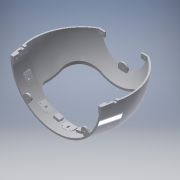
# Autodesk Inventor part: front
Saved by Autodesk Inventor 2017 (Build 210142000, 142)
## iProperties
Part Number: front
Material: Genérico
Document SubType Name: Modeling
Designer: Roberto
Density: 1 g/cm^3
Appearance: Valor por defecto
Author: Roberto
Autodesk Inventor part; units mm, degrees
ref_plane "XY Plane" through (0, 0, 0) normal (0, 0, 1) x (1, 0, 0)
sketch "Boceto1" plane through (0, 0, 0) normal (0, 0, 1) x (1, 0, 0)
  line L0 (-0.611288, 3.290752) -> (-0.374025, 3.347948)
  line L1 (0.276744, 0) -> (-0.374025, 3.347948)
  line L2 (-0.374025, 3.347945) -> (0.276744, 0)
  line L3 (-0.611288, 3.290752) -> (0, 0)
  line L4 (-0.611288, 3.290752) -> (0, 0)
  line L5 (0, 0) -> (0.3056, 0)
  line L6 (0.276744, 0) -> (0, 0)
  line L7 (0, 0) -> (0.3056, 0)
  line L8 (0, 0) -> (15, 0)
  arc A0 (3.961812, 11.346952) -> (-0.374025, 3.347948) centre (7.685812, 4.153752) ccw
  arc A1 (7.5, 12.385014) -> (3.894598, 11.311754) centre (8.396412, 2.781252) ccw
  line L9 (7.5, 12.627938) -> (7.5, 12.385014)
  arc A2 (7.5, 12.627938) -> (3.850449, 11.561628) centre (8.396412, 2.781252) ccw
  arc A3 (3.850449, 11.561628) -> (-0.611288, 3.290752) centre (7.685812, 4.153752) ccw
  line L10 (7.5, 0) -> (7.5, 18.610852)
  dimension "d0" = 15
  constraints: 22 end point, 11 point on circle, 4 centre point, 3 collinear, 3 horizontal, 2 coincident, 2 vertical, 1 midpoint
  measures "d0" distance of L5.start L8.end
revolve "Revolución1" add sketch "Boceto1" angle 180 about axis through (7.5, 12.627938, 0) along (0, -1, 0) contours A3 A2 L9 A1 A0 L0 | L0 L1 L5 L3
sketch "Boceto2" plane through (7.5, 0, 0) normal (0, -1, 0) x (1, 0, 0)
  circle A0 centre (-4.734, 4.734) radius 0.15
  circle A1 centre (4.734, 4.734) radius 0.15
  arc A2 (7.5, 0) -> (-7.5, 0) centre (0, 0) ccw
  arc A3 (-5.19458, 4.349466) -> (-4.349466, 5.19458) centre (-4.734, 4.734) ccw
  line L0 (-4.27342, 5.118534) -> (-4.763502, 5.608616)
  line L1 (-5.118534, 4.273421) -> (-5.611701, 4.766588)
  line L2 (0, 0) -> (0, 11.293859)
  circle A4 centre (4.734, 4.734) radius 0.15
  arc A5 (7.5, 0) -> (-7.5, 0) centre (0, 0) ccw
  arc A6 (4.349466, 5.19458) -> (5.19458, 4.349466) centre (4.734, 4.734) ccw
  line L3 (4.27342, 5.118534) -> (4.863883, 5.708997)
  line L4 (5.118534, 4.273421) -> (5.610829, 4.765715)
  line L5 (-4.663121, 5.508235) -> (-4.763502, 5.608616)
  line L6 (-5.514406, 4.669292) -> (-5.611701, 4.766588)
  line L7 (-5.611701, 4.766588) -> (-4.763502, 5.608616)
  arc A7 (7.223256, 0) -> (-7.223256, 0) centre (0, 0) ccw
  line L8 (5.512661, 4.667548) -> (5.610829, 4.765715)
  line L9 (4.667547, 5.512661) -> (4.765715, 5.610829)
  line L10 (4.765715, 5.610829) -> (5.610829, 4.765715)
  line L11 (0, -0.038021) -> (3.635109, -0.038021)
  circle A8 centre (4.734, -4.734) radius 0.1
  line L12 (4.27342, -5.118534) -> (4.765715, -5.610829)
  circle A9 centre (4.734, -4.734) radius 0.1
  arc A10 (5.19458, -4.349466) -> (4.349466, -5.19458) centre (4.734, -4.734) ccw
  line L13 (5.118534, -4.273421) -> (5.610829, -4.765715)
  line L14 (4.765715, -5.610829) -> (5.610829, -4.765715)
  circle A11 centre (-4.734, -4.734) radius 0.1
  line L15 (0, -0.076042) -> (0, -11.369902)
  arc A12 (-7.223256, 0) -> (7.223256, 0) centre (0, 0) ccw
  arc A13 (-7.5, 0) -> (7.5, 0) centre (0, 0) ccw
  line L16 (-4.27342, -5.118534) -> (-4.763502, -5.608616)
  arc A14 (-4.349466, -5.19458) -> (-5.19458, -4.349466) centre (-4.734, -4.734) ccw
  line L17 (-5.118534, -4.273421) -> (-5.611701, -4.766588)
  line L18 (-5.611701, -4.766588) -> (-4.763502, -5.608616)
  arc A15 (-7.5, 0) -> (7.5, 0) centre (0, 0) ccw
  line L19 (0, -7.5) -> (0.400854, -7.674504)
  line L20 (0, -7.576042) -> (0.142839, -7.719539)
  point P0 (-4.863883, 5.708997)
  point P1 (-5.708996, 4.863883)
  point P2 (5.708996, 4.863883)
  point P3 (5.708996, -4.939925)
  point P4 (-4.863883, -5.785039)
  point P5 (-5.708996, -4.939925)
  dimension "d2" = 1.2
  dimension "d120" = 0.2
  dimension "d121" = 0.2
  dimension "d122" = 0.2
  constraints: 42 end point, 25 point on circle, 15 centre point, 14 symmetric about line, 13 point on line, 4 coincident, 2 parallel, 1 collinear, 1 horizontal, 1 vertical, 3 other
  measures "d2" diameter of A3
  measures "d120" diameter of A11
  measures "d121" diameter of A8
  measures "d122" diameter of A9
extrude "Extrusión1" add sketch "Boceto2" against normal blind 0.3 contours L16 L18 L17 A12 | A12 L17 A14 L16 | A12 L13 L14 L12 | L12 A10 L13 A12
sketch "Boceto3" plane through (7.685812, 4.153752, 0) normal (0, 0, 1) x (0.8801071, -0.4747751, 0)
  line L0 (-2.299378, -5.960001) -> (5.916505, -1.52793)
  line L1 (2.389364, 0.225418) -> (0.289514, -0.927498)
  line L2 (-4.303117, -3.404512) -> (0.289514, -0.927498)
  line L3 (8.166085, -0.315066) -> (-4.548958, -7.172866)
  line L4 (4.675509, 1.458439) -> (2.575659, 0.305524)
  arc A0 (4.675509, 1.458439) -> (5.077156, 2.950396) centre (4.160061, 2.397244) ccw
  arc A1 (3.665081, 5.291538) -> (-1.111974, 6.051545) centre (0.856861, 3.03355) ccw
  line L5 (3.665081, 5.291538) -> (5.077156, 2.950396)
  line L6 (-4.792767, 4.066326) -> (-1.111974, 6.051545)
  line L7 (-3.075408, -2.732168) -> (3.625584, 0.881981)
  line L8 (-2.016972, -2.171491) -> (2.575659, 0.305524)
  arc A2 (-5.601178, -2.808914) -> (-4.133845, -3.292845) centre (-4.635182, -2.34643) ccw
  line L9 (-6.781799, -0.342939) -> (-5.601178, -2.808914)
  arc A3 (-4.792767, 4.066326) -> (-6.781799, -0.342939) centre (-3.352393, 0.763308) ccw
  line L10 (-4.792533, -7.304237) -> (-1.647022, -5.607386)
  line L11 (1.808563, -3.743966) -> (5.744335, -10.648473)
  line L12 (-4.133845, -3.292845) -> (4.675509, 1.458439)
  line L13 (-4.792767, 4.066326) -> (-1.111974, 6.051545)
  line L14 (-5.601178, -2.808914) -> (-6.781799, -0.342939)
  line L15 (5.077156, 2.950396) -> (3.665081, 5.291538)
  line L16 (-4.79224, -7.304779) -> (8.409367, -0.183152)
  line L17 (1.808563, -3.743966) -> (1.713623, -3.567937)
  dimension "d167" = 0.2
  constraints: 32 end point, 8 point on circle, 4 centre point, 3 midpoint, 2 parallel, 1 collinear, 1 perpendicular, 1 point on line
  measures "d167" distance of L17.start L17.end
extrude "Extrusión2" cut sketch "Boceto3" against normal blind 10 contours L12 A2 L9 A3 L6 A1 L5 A0
sketch "Boceto4" plane through (7.685812, 4.153752, 0) normal (0, 0, 1) x (0.8801071, -0.4747751, 0)
  line L0 (7.149027, 2.940979) -> (8.165803, -0.314543)
  line L1 (8.165803, -0.314543) -> (8.409367, -0.183152)
  line L2 (8.409367, -0.183152) -> (7.384998, 3.003286)
  arc A0 (7.384998, 3.003286) -> (-0.468614, 8.164221) centre (-0.32707, -0.176438) ccw
  arc A1 (-0.468614, 8.164221) -> (-4.186868, 7.369973) centre (-0.300845, -1.72176) ccw
  arc A2 (-4.186868, 7.369973) -> (-6.892606, 4.698789) centre (1.277033, -0.870572) ccw
  arc A3 (-6.892606, 4.698789) -> (-6.892606, -4.698789) centre (0, 0) ccw
  line L3 (-6.892606, -4.698789) -> (-4.79224, -7.304779)
  line L4 (-4.79224, -7.304779) -> (-4.548676, -7.173388)
  line L5 (-4.548676, -7.173388) -> (-6.710945, -4.535804)
  arc A4 (-6.735116, 4.499834) -> (-6.710945, -4.535804) centre (0, 0) ccw
  arc A5 (-4.071533, 7.156173) -> (-6.735116, 4.499834) centre (1.277033, -0.870572) ccw
  arc A6 (-0.388836, 7.923345) -> (-4.071533, 7.156173) centre (-0.300845, -1.72176) ccw
  arc A7 (7.149027, 2.940979) -> (-0.388836, 7.923345) centre (-0.32707, -0.176438) ccw
extrude "Extrusión3" add sketch "Boceto4" along normal blind 0.1
ref_plane "Plano de trabajo1" through (7.5, 0, 0) normal (1, 0, 0) x (0, 1, 0)
ref_plane "Plano de trabajo2" through (0, 2, 0) normal (0, 1, 0) x (-1, 0, 0)
sketch "Boceto6" plane through (0, 2, 0) normal (0, 1, 0) x (-1, 0, 0)
  line L0 (-15, 0.1) -> (-15.611288, 0.1)
  line L1 (-0.381713, -3.084014) -> (-1.270022, -4.622611)
  line L2 (-1.270022, -4.622611) -> (-1.486529, -4.497611)
  line L3 (-4.540986, -6.901781) -> (-3.002389, -6.013471)
  line L4 (-2.877389, -6.229978) -> (-3.002389, -6.013471)
  line L5 (0.206624, -0.888309) -> (-0.043376, -0.888309)
  line L6 (-0.381713, -3.084014) -> (-0.598219, -2.959014)
  line L7 (-6.611691, -7.706624) -> (-8.388309, -7.706624)
  line L8 (-8.388309, -7.706624) -> (-8.388309, -7.456624)
  line L9 (-1.486529, -4.497611) -> (-0.598219, -2.959014)
  line L10 (-2.877389, -6.229978) -> (-4.415986, -7.118287)
  line L11 (-4.415986, -7.118287) -> (-4.540986, -6.901781)
  line L12 (-8.388309, -7.456624) -> (-6.611691, -7.456624)
  line L13 (-6.611691, -7.706624) -> (-6.611691, -7.456624)
  line L14 (-0.276744, 0.1) -> (0.374025, 0.1)
  line L15 (0.206624, -0.888309) -> (-0.043376, -0.888309)
  line L16 (-0.043376, -0.888309) -> (-0.043376, 0.1)
  line L17 (-0.043376, 0.1) -> (0.206624, 0.1)
  line L18 (0.206624, 0.1) -> (0.206624, -0.888309)
  line L19 (-7.5, 0) -> (-7.5, -4.175749)
  line L20 (-14.618287, -3.084014) -> (-13.729978, -4.622611)
  line L21 (-13.729978, -4.622611) -> (-13.513471, -4.497611)
  line L22 (-10.459014, -6.901781) -> (-11.997611, -6.013471)
  line L23 (-12.122611, -6.229978) -> (-11.997611, -6.013471)
  line L24 (-15.206624, -0.888309) -> (-14.956624, -0.888309)
  line L25 (-14.618287, -3.084014) -> (-14.401781, -2.959014)
  line L26 (-13.513471, -4.497611) -> (-14.401781, -2.959014)
  line L27 (-12.122611, -6.229978) -> (-10.584014, -7.118287)
  line L28 (-10.584014, -7.118287) -> (-10.459014, -6.901781)
  line L29 (-14.723256, 0.1) -> (-15.374025, 0.1)
  line L30 (-15.206624, -0.888309) -> (-14.956624, -0.888309)
  line L31 (-14.956624, -0.888309) -> (-14.956624, 0.1)
  line L32 (-14.956624, 0.1) -> (-15.206624, 0.1)
  line L33 (-15.206624, 0.1) -> (-15.206624, -0.888309)
  line L34 (-6.611691, -7.706624) -> (-8.388309, -7.706624)
  line L35 (-8.388309, -7.706624) -> (-8.388309, -7.456624)
  line L36 (-8.388309, -7.456624) -> (-6.611691, -7.456624)
  line L37 (-6.611691, -7.456624) -> (-6.611691, -7.706624)
  line L38 (-2.877389, -6.229978) -> (-3.002389, -6.013471)
  line L39 (-2.877389, -6.229978) -> (-4.415986, -7.118287)
  line L40 (-4.415986, -7.118287) -> (-4.540986, -6.901781)
  line L41 (-4.540986, -6.901781) -> (-3.002389, -6.013471)
  line L42 (-10.584014, -7.118287) -> (-12.122611, -6.229978)
  line L43 (-12.122611, -6.229978) -> (-11.997611, -6.013471)
  line L44 (-11.997611, -6.013471) -> (-10.459014, -6.901781)
  line L45 (-10.459014, -6.901781) -> (-10.584014, -7.118287)
  line L46 (-13.513471, -4.497611) -> (-13.729978, -4.622611)
  line L47 (-13.729978, -4.622611) -> (-14.618287, -3.084014)
  line L48 (-14.618287, -3.084014) -> (-14.401781, -2.959014)
  line L49 (-14.401781, -2.959014) -> (-13.513471, -4.497611)
  line L50 (-15.206624, 0.1) -> (-14.956624, 0.1)
  line L51 (-14.956624, 0.1) -> (-14.956624, -0.888309)
  line L52 (-14.956624, -0.888309) -> (-15.206624, -0.888309)
  line L53 (-15.206624, -0.888309) -> (-15.206624, 0.1)
  line L54 (-2.877389, -6.229978) -> (-3.002389, -6.013471)
  line L55 (-4.415986, -7.118287) -> (-2.877389, -6.229978)
  line L56 (-3.002389, -6.013471) -> (-4.540986, -6.901781)
  line L57 (-4.540986, -6.901781) -> (-4.415986, -7.118287)
  line L58 (-0.381713, -3.084014) -> (-0.598219, -2.959014)
  line L59 (-0.598219, -2.959014) -> (-1.486529, -4.497611)
  line L60 (-1.486529, -4.497611) -> (-1.270022, -4.622611)
  line L61 (-1.270022, -4.622611) -> (-0.381713, -3.084014)
  line L62 (0.206624, -0.888309) -> (0.206624, 0.1)
  line L63 (0.206624, 0.1) -> (-0.043376, 0.1)
  line L64 (-0.043376, 0.1) -> (-0.043376, -0.888309)
  line L65 (-0.043376, -0.888309) -> (0.206624, -0.888309)
  line L66 (-7.5, -7.456624) -> (-7.5, -6.737352)
  line L67 (-6.131323, -6.846637) -> (-5.987048, -7.38508)
  line L68 (-5.26199, -6.6137) -> (-5.117715, -7.152143)
  line L69 (-6.131323, -6.846637) -> (-5.26199, -6.6137)
  line L70 (-5.987048, -7.38508) -> (-5.117715, -7.152143)
  circle A0 centre (-5.624519, -6.99939) radius 0.1
  line L71 (-8.868677, -6.846637) -> (-9.012952, -7.38508)
  line L72 (-9.73801, -6.6137) -> (-9.882285, -7.152143)
  line L73 (-8.868677, -6.846637) -> (-9.73801, -6.6137)
  line L74 (-9.012952, -7.38508) -> (-9.882285, -7.152143)
  circle A1 centre (-9.375481, -6.99939) radius 0.1
  point P0 (0, 0)
  point P1 (-15, 0)
  dimension "d13" = 0.25
  dimension "d18" = 0.25
  dimension "d19" = 0.25
  dimension "d20" = 0.25
  dimension "d170" = 0.2
  constraints: 146 end point, 26 symmetric about line, 20 perpendicular, 9 parallel, 5 collinear, 4 horizontal, 2 centre point, 2 point on line, 2 vertical, 1 midpoint, 1 other
  measures "d13" distance of L2.end L1.end
  measures "d18" distance of L5.start L5.end
  measures "d19" distance of L8.end L7.end
  measures "d20" distance of L10.end L11.end
  measures "d170" diameter of A0
extrude "Extrusión4" add sketch "Boceto6" along normal blind 0.735 and the other way blind 0.535 contours L29 L31 L24 L33 L0 | L1 L2 L9 L6 | L3 L4 L10 L11 | L5 L16 L14 L18 | L7 L8 L12 L13 | L25 L26 L21 L20 | L28 L27 L23 L22
sketch "Boceto8" plane through (6.611691, 2.735, -7.456624) normal (0, 0, 1) x (1, 0, 0)
  line L0 (1.78, 0) -> (1.78, -1.27)
  line L1 (1.012029, -0.460231) -> (0.772029, -0.460231)
  line L2 (0.772029, -0.460231) -> (0.772029, -0.910231)
  line L3 (0.772029, -0.910231) -> (1.012029, -0.910231)
  line L4 (1.012029, -0.910231) -> (1.012029, -0.460231)
  line L5 (1.78, 0) -> (0, 0)
  line L6 (0, 0) -> (0, -1.27)
  line L7 (0, -1.27) -> (1.78, -1.27)
  line L8 (1.78, -1.27) -> (1.78, -1.02)
  circle A0 centre (1.53, -1.02) radius 0.075
  line L9 (1.78, 0) -> (1.78, -0.12)
  circle A1 centre (1.66, -0.12) radius 0.06
  circle A2 centre (1.4, -0.12) radius 0.06
  circle A3 centre (1.14, -0.12) radius 0.06
  circle A4 centre (0.88, -0.12) radius 0.06
  circle A5 centre (0.62, -0.12) radius 0.06
  circle A6 centre (0.12, -0.12) radius 0.06
  circle A7 centre (0.38, -0.12) radius 0.06
  line L10 (1.604331, -0.280161) -> (1.464331, -0.280161)
  line L11 (1.464331, -0.280161) -> (1.464331, -0.580161)
  line L12 (1.464331, -0.580161) -> (1.604331, -0.580161)
  line L13 (1.604331, -0.580161) -> (1.604331, -0.280161)
  circle A8 centre (0.25, -1.02) radius 0.075
  point P0 (-6.611691, -2.735)
  dimension "d21" = 1.78
  dimension "d22" = 1.27
  dimension "d132" = 0.15
  dimension "d133" = 0.15
  constraints: 28 end point, 9 centre point, 2 point on line
  measures "d21" distance of L6.end L0.end
  measures "d22" distance of L6.start L6.end
  measures "d132" diameter of A8
  measures "d133" diameter of A0
sketch "Boceto9" plane through (4.540986, 1.47184, -6.901781) normal (0.5, 0, 0.8660254) x (0.8660254, 0, -0.5)
  circle A0 centre (-0.116619, 1.14316) radius 0.06
  line L0 (0.003381, 1.26316) -> (0.003381, 1.14316)
  line L1 (-0.172288, 0.983) -> (-0.312288, 0.983)
  circle A1 centre (-1.156619, 1.14316) radius 0.06
  circle A2 centre (-1.526619, 0.24316) radius 0.075
  line L2 (-1.776619, 1.26316) -> (-1.776619, -0.00684)
  circle A3 centre (-1.396619, 1.14316) radius 0.06
  circle A4 centre (-1.656619, 1.14316) radius 0.06
  circle A5 centre (-0.376619, 1.14316) radius 0.06
  line L3 (-0.312288, 0.983) -> (-0.312288, 0.683)
  line L4 (-0.172288, 0.683) -> (-0.172288, 0.983)
  line L5 (-0.312288, 0.683) -> (-0.172288, 0.683)
  circle A6 centre (-0.636619, 1.14316) radius 0.06
  circle A7 centre (-0.896619, 1.14316) radius 0.06
  circle A8 centre (-0.246619, 0.24316) radius 0.075
  line L6 (0.003381, 1.26316) -> (0.003381, -0.00684)
  line L7 (0.003381, -0.00684) -> (0.003381, 0.24316)
  line L8 (0.003381, 1.26316) -> (-1.776619, 1.26316)
  line L9 (-1.776619, -0.00684) -> (0.003381, -0.00684)
  line L10 (-0.76459, 0.802929) -> (-1.00459, 0.802929)
  line L11 (-0.76459, 0.352929) -> (-0.76459, 0.802929)
  line L12 (-1.00459, 0.352929) -> (-0.76459, 0.352929)
  line L13 (-1.00459, 0.802929) -> (-1.00459, 0.352929)
  point P0 (-7.3835, -1.47184)
  dimension "d23" = 1.78
  dimension "d24" = 1.27
  dimension "d134" = 0.15
  dimension "d135" = 0.15
  constraints: 28 end point, 9 centre point, 2 point on line
  measures "d23" distance of L9.start L7.start
  measures "d24" distance of L8.end L9.start
  measures "d134" diameter of A8
  measures "d135" diameter of A2
sketch "Boceto10" plane through (1.486529, 1.47184, -4.497611) normal (0.8660254, 0, 0.5) x (0.5, 0, -0.8660254)
  line L0 (0.003381, -0.00684) -> (0.003381, 0.24316)
  line L1 (-0.312288, 0.683) -> (-0.172288, 0.683)
  line L2 (-0.172288, 0.683) -> (-0.172288, 0.983)
  line L3 (-0.172288, 0.983) -> (-0.312288, 0.983)
  line L4 (-0.312288, 0.983) -> (-0.312288, 0.683)
  line L5 (-1.00459, 0.352929) -> (-0.76459, 0.352929)
  line L6 (-0.76459, 0.352929) -> (-0.76459, 0.802929)
  line L7 (0.003381, 1.26316) -> (0.003381, -0.00684)
  line L8 (-0.76459, 0.802929) -> (-1.00459, 0.802929)
  line L9 (-1.00459, 0.802929) -> (-1.00459, 0.352929)
  line L10 (-1.776619, -0.00684) -> (0.003381, -0.00684)
  circle A0 centre (-0.376619, 1.14316) radius 0.06
  circle A1 centre (-0.636619, 1.14316) radius 0.06
  circle A2 centre (-0.896619, 1.14316) radius 0.06
  line L11 (0.003381, 1.26316) -> (-1.776619, 1.26316)
  circle A3 centre (-1.156619, 1.14316) radius 0.06
  circle A4 centre (-0.116619, 1.14316) radius 0.06
  line L12 (0.003381, 1.26316) -> (0.003381, 1.14316)
  circle A5 centre (-1.526619, 0.24316) radius 0.075
  circle A6 centre (-1.396619, 1.14316) radius 0.06
  circle A7 centre (-1.656619, 1.14316) radius 0.06
  line L13 (-1.776619, 1.26316) -> (-1.776619, -0.00684)
  circle A8 centre (-0.246619, 0.24316) radius 0.075
  point P0 (-4.638309, -1.47184)
  dimension "d25" = 1.78
  dimension "d26" = 1.27
  dimension "d136" = 0.15
  dimension "d137" = 0.15
  constraints: 28 end point, 9 centre point, 2 point on line
  measures "d25" distance of L10.start L0.start
  measures "d26" distance of L11.end L10.start
  measures "d136" diameter of A8
  measures "d137" diameter of A5
sketch "Boceto11" plane through (11.997611, 1.47184, -6.013471) normal (-0.5, 0, 0.8660254) x (0.8660254, 0, 0.5)
  line L0 (0.003381, -0.00684) -> (0.003381, 0.24316)
  line L1 (-0.312288, 0.683) -> (-0.172288, 0.683)
  line L2 (-0.172288, 0.683) -> (-0.172288, 0.983)
  line L3 (-0.172288, 0.983) -> (-0.312288, 0.983)
  line L4 (-0.312288, 0.983) -> (-0.312288, 0.683)
  line L5 (-1.00459, 0.352929) -> (-0.76459, 0.352929)
  line L6 (-0.76459, 0.352929) -> (-0.76459, 0.802929)
  line L7 (0.003381, 1.26316) -> (0.003381, -0.00684)
  line L8 (-0.76459, 0.802929) -> (-1.00459, 0.802929)
  line L9 (-1.00459, 0.802929) -> (-1.00459, 0.352929)
  line L10 (-1.776619, -0.00684) -> (0.003381, -0.00684)
  circle A0 centre (-0.376619, 1.14316) radius 0.06
  circle A1 centre (-0.636619, 1.14316) radius 0.06
  circle A2 centre (-0.896619, 1.14316) radius 0.06
  line L11 (0.003381, 1.26316) -> (-1.776619, 1.26316)
  circle A3 centre (-1.156619, 1.14316) radius 0.06
  circle A4 centre (-0.116619, 1.14316) radius 0.06
  line L12 (0.003381, 1.26316) -> (0.003381, 1.14316)
  circle A5 centre (-1.526619, 0.24316) radius 0.075
  circle A6 centre (-1.396619, 1.14316) radius 0.06
  circle A7 centre (-1.656619, 1.14316) radius 0.06
  line L13 (-1.776619, 1.26316) -> (-1.776619, -0.00684)
  circle A8 centre (-0.246619, 0.24316) radius 0.075
  point P0 (-7.3835, -1.47184)
  dimension "d27" = 1.78
  dimension "d28" = 1.27
  dimension "d130" = 0.15
  dimension "d131" = 0.15
  constraints: 28 end point, 9 centre point, 2 point on line
  measures "d27" distance of L10.start L0.start
  measures "d28" distance of L11.end L10.start
  measures "d130" diameter of A5
  measures "d131" diameter of A8
sketch "Boceto12" plane through (14.401781, 1.47184, -2.959014) normal (-0.8660254, 0, 0.5) x (0.5, 0, 0.8660254)
  line L0 (0.003381, -0.00684) -> (0.003381, 0.24316)
  line L1 (-0.312288, 0.683) -> (-0.172288, 0.683)
  line L2 (-0.172288, 0.683) -> (-0.172288, 0.983)
  line L3 (-0.172288, 0.983) -> (-0.312288, 0.983)
  line L4 (-0.312288, 0.983) -> (-0.312288, 0.683)
  line L5 (-1.00459, 0.352929) -> (-0.76459, 0.352929)
  line L6 (-0.76459, 0.352929) -> (-0.76459, 0.802929)
  line L7 (0.003381, 1.26316) -> (0.003381, -0.00684)
  line L8 (-0.76459, 0.802929) -> (-1.00459, 0.802929)
  line L9 (-1.00459, 0.802929) -> (-1.00459, 0.352929)
  line L10 (-1.776619, -0.00684) -> (0.003381, -0.00684)
  circle A0 centre (-0.376619, 1.14316) radius 0.06
  circle A1 centre (-0.636619, 1.14316) radius 0.06
  circle A2 centre (-0.896619, 1.14316) radius 0.06
  line L11 (0.003381, 1.26316) -> (-1.776619, 1.26316)
  circle A3 centre (-1.156619, 1.14316) radius 0.06
  circle A4 centre (-0.116619, 1.14316) radius 0.06
  line L12 (0.003381, 1.26316) -> (0.003381, 1.14316)
  circle A5 centre (-1.526619, 0.24316) radius 0.075
  circle A6 centre (-1.396619, 1.14316) radius 0.06
  circle A7 centre (-1.656619, 1.14316) radius 0.06
  line L13 (-1.776619, 1.26316) -> (-1.776619, -0.00684)
  circle A8 centre (-0.246619, 0.24316) radius 0.075
  point P0 (-4.638309, -1.47184)
  dimension "d29" = 1.78
  dimension "d30" = 1.27
  dimension "d128" = 0.15
  dimension "d129" = 0.15
  constraints: 28 end point, 9 centre point, 2 point on line
  measures "d29" distance of L10.start L0.start
  measures "d30" distance of L11.end L10.start
  measures "d128" diameter of A8
  measures "d129" diameter of A5
sketch "Boceto13" plane through (14.956624, 1.465, 0.1) normal (-1, 0, 0) x (0, 0, 1)
  line L0 (0.791691, 0) -> (0.791691, 0.25)
  line L1 (0.476022, 0.689839) -> (0.616022, 0.689839)
  line L2 (0.616022, 0.689839) -> (0.616022, 0.989839)
  line L3 (0.616022, 0.989839) -> (0.476022, 0.989839)
  line L4 (0.476022, 0.989839) -> (0.476022, 0.689839)
  line L5 (-0.21628, 0.359769) -> (0.02372, 0.359769)
  line L6 (0.02372, 0.359769) -> (0.02372, 0.809769)
  line L7 (0.791691, 1.27) -> (0.791691, 0)
  line L8 (0.02372, 0.809769) -> (-0.21628, 0.809769)
  line L9 (-0.21628, 0.809769) -> (-0.21628, 0.359769)
  line L10 (-0.988309, 0) -> (0.791691, 0)
  circle A0 centre (0.411691, 1.15) radius 0.06
  circle A1 centre (0.151691, 1.15) radius 0.06
  circle A2 centre (-0.108309, 1.15) radius 0.06
  line L11 (0.791691, 1.27) -> (-0.988309, 1.27)
  circle A3 centre (-0.368309, 1.15) radius 0.06
  circle A4 centre (0.671691, 1.15) radius 0.06
  line L12 (0.791691, 1.27) -> (0.791691, 1.15)
  circle A5 centre (-0.738309, 0.25) radius 0.075
  circle A6 centre (-0.608309, 1.15) radius 0.06
  circle A7 centre (-0.868309, 1.15) radius 0.06
  line L13 (-0.988309, 1.27) -> (-0.988309, 0)
  circle A8 centre (0.541691, 0.25) radius 0.11
  line L14 (-0.988309, 1.27) -> (0, 1.27)
  line L15 (0, 1.27) -> (0, 0)
  line L16 (0, 1.27) -> (0.791691, 1.27)
  line L17 (0.791691, 1.27) -> (0.791691, 0)
  line L18 (0.791691, 0) -> (0, 0)
  line L19 (0, 0) -> (0, 1.27)
  line L20 (0, -1.465) -> (1.766659, -1.465)
  line L21 (0, 0) -> (0, -1.465)
  point P0 (-0.1, -1.465)
  dimension "d31" = 1.78
  dimension "d32" = 1.27
  dimension "d127" = 0.15
  constraints: 42 end point, 9 centre point, 3 point on line, 2 horizontal, 2 parallel, 2 perpendicular, 1 vertical
  measures "d31" distance of L10.start L0.start
  measures "d32" distance of L11.end L10.start
  measures "d127" diameter of A5
sketch "Boceto14" plane through (0.043376, 1.465, 0.1) normal (1, 0, 0) x (0, 0, -1)
  line L0 (0.988309, 0.00684) -> (0.988309, 1.27)
  line L1 (0.976999, 0) -> (0.1, 0)
  line L2 (-0.02372, 0.359769) -> (-0.02372, 0.809769)
  line L3 (0.21628, 0.809769) -> (0.21628, 0.359769)
  line L4 (-0.02372, 0.809769) -> (0.21628, 0.809769)
  line L5 (0.21628, 0.359769) -> (-0.02372, 0.359769)
  circle A0 centre (0.738309, 0.25) radius 0.075
  circle A1 centre (-0.541691, 0.25) radius 0.11
  line L6 (-0.791691, 1.27) -> (-0.791691, 0)
  point P0 (0.1, -1.465)
  dimension "d123" = 0.15
  measures "d123" diameter of A0
extrude "Extrusión5" cut sketch "Boceto14" against normal blind 0.15 contours A0
extrude "Extrusión6" cut sketch "Boceto10" against normal blind 0.15 contours A5 | A8
extrude "Extrusión7" cut sketch "Boceto9" against normal blind 0.15 contours A2 | A8
extrude "Extrusión8" cut sketch "Boceto8" against normal blind 0.15 contours A0 | A8
extrude "Extrusión9" cut sketch "Boceto11" against normal blind 0.15 contours A5 | A8
extrude "Extrusión10" cut sketch "Boceto12" against normal blind 0.15 contours A5 | A8
extrude "Extrusión11" cut sketch "Boceto13" against normal blind 0.15 contours A5
sketch "Boceto15" plane through (14.956624, 1.465, 0.1) normal (-1, 0, 0) x (0, 0, 1)
  line L0 (0.616022, 0.989839) -> (0.476022, 0.989839)
  line L1 (0.476022, 0.689839) -> (0.616022, 0.689839)
  line L2 (0.616022, 0.689839) -> (0.616022, 0.989839)
  circle A0 centre (0.671691, 1.15) radius 0.06
  line L3 (0.791691, 1.27) -> (0.791691, 1.15)
  line L4 (0.476022, 0.989839) -> (0.476022, 0.689839)
  line L5 (0.791691, 0) -> (0.791691, 0.25)
  circle A1 centre (0.411691, 1.15) radius 0.06
  circle A2 centre (0.151691, 1.15) radius 0.06
  circle A3 centre (-0.108309, 1.15) radius 0.06
  line L6 (0.02372, 0.809769) -> (-0.21628, 0.809769)
  circle A4 centre (0.541691, 0.25) radius 0.11
  line L7 (0.02372, 0.359769) -> (0.02372, 0.809769)
  line L8 (0.791691, 1.27) -> (0.791691, 0)
  circle A5 centre (-0.368309, 1.15) radius 0.06
  line L9 (-0.21628, 0.359769) -> (0.02372, 0.359769)
  line L10 (-0.21628, 0.809769) -> (-0.21628, 0.359769)
  line L11 (0.791691, 1.27) -> (-0.988309, 1.27)
  line L12 (-0.988309, 0) -> (0.791691, 0)
  line L13 (-0.988309, 1.27) -> (-0.988309, 0)
  circle A6 centre (-0.608309, 1.15) radius 0.06
  circle A7 centre (-0.868309, 1.15) radius 0.06
  circle A8 centre (-0.738309, 0.25) radius 0.11
  point P0 (-0.1, -1.465)
  dimension "d47" = 1.78
  dimension "d48" = 1.27
  constraints: 28 end point, 9 centre point, 2 point on line
  measures "d47" distance of L12.start L8.end
  measures "d48" distance of L11.end L12.start
extrude "Extrusión12" cut sketch "Boceto15" against normal blind 15 contours L7 L9 L10 L6
sketch "Boceto16" plane through (14.401781, 1.47184, -2.959014) normal (-0.8660254, 0, 0.5) x (0.5, 0, 0.8660254)
  line L0 (-0.172288, 0.983) -> (-0.312288, 0.983)
  line L1 (-0.312288, 0.683) -> (-0.172288, 0.683)
  line L2 (-0.172288, 0.683) -> (-0.172288, 0.983)
  circle A0 centre (-0.116619, 1.14316) radius 0.06
  line L3 (0.003381, 1.26316) -> (0.003381, 1.14316)
  line L4 (-0.312288, 0.983) -> (-0.312288, 0.683)
  line L5 (0.003381, -0.00684) -> (0.003381, 0.24316)
  circle A1 centre (-0.376619, 1.14316) radius 0.06
  circle A2 centre (-0.636619, 1.14316) radius 0.06
  circle A3 centre (-0.896619, 1.14316) radius 0.06
  line L6 (-0.76459, 0.802929) -> (-1.00459, 0.802929)
  circle A4 centre (-0.246619, 0.24316) radius 0.11
  line L7 (-0.76459, 0.352929) -> (-0.76459, 0.802929)
  line L8 (0.003381, 1.26316) -> (0.003381, -0.00684)
  circle A5 centre (-1.156619, 1.14316) radius 0.06
  line L9 (-1.00459, 0.352929) -> (-0.76459, 0.352929)
  line L10 (-1.00459, 0.802929) -> (-1.00459, 0.352929)
  line L11 (0.003381, 1.26316) -> (-1.776619, 1.26316)
  line L12 (-1.776619, -0.00684) -> (0.003381, -0.00684)
  line L13 (-1.776619, 1.26316) -> (-1.776619, -0.00684)
  circle A6 centre (-1.396619, 1.14316) radius 0.06
  circle A7 centre (-1.656619, 1.14316) radius 0.06
  circle A8 centre (-1.526619, 0.24316) radius 0.11
  point P0 (-4.638309, -1.47184)
  dimension "d51" = 1.78
  dimension "d52" = 1.27
  constraints: 28 end point, 9 centre point, 2 point on line
  measures "d51" distance of L12.start L12.end
  measures "d52" distance of L11.end L12.start
extrude "Extrusión13" cut sketch "Boceto16" against normal blind 15 contours L7 L9 L10 L6
sketch "Boceto17" plane through (11.997611, 1.47184, -6.013471) normal (-0.5, 0, 0.8660254) x (0.8660254, 0, 0.5)
  line L0 (-0.172288, 0.983) -> (-0.312288, 0.983)
  line L1 (-0.312288, 0.683) -> (-0.172288, 0.683)
  line L2 (-0.172288, 0.683) -> (-0.172288, 0.983)
  circle A0 centre (-0.116619, 1.14316) radius 0.06
  line L3 (0.003381, 1.26316) -> (0.003381, 1.14316)
  line L4 (-0.312288, 0.983) -> (-0.312288, 0.683)
  line L5 (0.003381, -0.00684) -> (0.003381, 0.24316)
  circle A1 centre (-0.376619, 1.14316) radius 0.06
  circle A2 centre (-0.636619, 1.14316) radius 0.06
  circle A3 centre (-0.896619, 1.14316) radius 0.06
  line L6 (-0.76459, 0.802929) -> (-1.00459, 0.802929)
  circle A4 centre (-0.246619, 0.24316) radius 0.11
  line L7 (-0.76459, 0.352929) -> (-0.76459, 0.802929)
  line L8 (0.003381, 1.26316) -> (0.003381, -0.00684)
  circle A5 centre (-1.156619, 1.14316) radius 0.06
  line L9 (-1.00459, 0.352929) -> (-0.76459, 0.352929)
  line L10 (-1.00459, 0.802929) -> (-1.00459, 0.352929)
  line L11 (0.003381, 1.26316) -> (-1.776619, 1.26316)
  line L12 (-1.776619, -0.00684) -> (0.003381, -0.00684)
  line L13 (-1.776619, 1.26316) -> (-1.776619, -0.00684)
  circle A6 centre (-1.396619, 1.14316) radius 0.06
  circle A7 centre (-1.656619, 1.14316) radius 0.06
  circle A8 centre (-1.526619, 0.24316) radius 0.11
  point P0 (-7.3835, -1.47184)
  dimension "d55" = 1.78
  dimension "d56" = 1.27
  constraints: 28 end point, 9 centre point, 2 point on line
  measures "d55" distance of L12.start L12.end
  measures "d56" distance of L11.end L12.start
extrude "Extrusión14" cut sketch "Boceto17" against normal blind 15 contours L7 L9 L10 L6
sketch "Boceto18" plane through (6.611691, 2.735, -7.456624) normal (0, 0, 1) x (1, 0, 0)
  circle A0 centre (1.66, -0.12) radius 0.06
  line L0 (1.78, 0) -> (1.78, -0.12)
  line L1 (1.604331, -0.280161) -> (1.464331, -0.280161)
  circle A1 centre (0.62, -0.12) radius 0.06
  circle A2 centre (0.25, -1.02) radius 0.11
  line L2 (0, 0) -> (0, -1.27)
  circle A3 centre (0.38, -0.12) radius 0.06
  circle A4 centre (0.12, -0.12) radius 0.06
  circle A5 centre (1.4, -0.12) radius 0.06
  line L3 (1.464331, -0.280161) -> (1.464331, -0.580161)
  line L4 (1.604331, -0.580161) -> (1.604331, -0.280161)
  line L5 (1.464331, -0.580161) -> (1.604331, -0.580161)
  circle A6 centre (1.14, -0.12) radius 0.06
  circle A7 centre (0.88, -0.12) radius 0.06
  circle A8 centre (1.53, -1.02) radius 0.11
  line L6 (1.78, 0) -> (1.78, -1.27)
  line L7 (1.78, -1.27) -> (1.78, -1.02)
  line L8 (1.78, 0) -> (0, 0)
  line L9 (0, -1.27) -> (1.78, -1.27)
  line L10 (1.012029, -0.460231) -> (0.772029, -0.460231)
  line L11 (1.012029, -0.910231) -> (1.012029, -0.460231)
  line L12 (0.772029, -0.910231) -> (1.012029, -0.910231)
  line L13 (0.772029, -0.460231) -> (0.772029, -0.910231)
  point P0 (-6.611691, -2.735)
  dimension "d59" = 1.78
  dimension "d60" = 1.27
  constraints: 28 end point, 9 centre point, 2 point on line
  measures "d59" distance of L9.start L6.end
  measures "d60" distance of L8.end L9.start
extrude "Extrusión15" cut sketch "Boceto18" against normal blind 15 contours L11 L12 L13 L10
sketch "Boceto19" plane through (4.540986, 1.47184, -6.901781) normal (0.5, 0, 0.8660254) x (0.8660254, 0, -0.5)
  line L0 (0.003381, -0.00684) -> (0.003381, 0.24316)
  line L1 (-0.312288, 0.683) -> (-0.172288, 0.683)
  line L2 (-0.172288, 0.683) -> (-0.172288, 0.983)
  line L3 (-0.172288, 0.983) -> (-0.312288, 0.983)
  line L4 (-0.312288, 0.983) -> (-0.312288, 0.683)
  line L5 (-1.00459, 0.352929) -> (-0.76459, 0.352929)
  line L6 (-0.76459, 0.352929) -> (-0.76459, 0.802929)
  line L7 (0.003381, 1.26316) -> (0.003381, -0.00684)
  line L8 (-0.76459, 0.802929) -> (-1.00459, 0.802929)
  line L9 (-1.00459, 0.802929) -> (-1.00459, 0.352929)
  line L10 (-1.776619, -0.00684) -> (0.003381, -0.00684)
  circle A0 centre (-0.376619, 1.14316) radius 0.06
  circle A1 centre (-0.636619, 1.14316) radius 0.06
  circle A2 centre (-0.896619, 1.14316) radius 0.06
  line L11 (0.003381, 1.26316) -> (-1.776619, 1.26316)
  circle A3 centre (-1.156619, 1.14316) radius 0.06
  circle A4 centre (-0.116619, 1.14316) radius 0.06
  line L12 (0.003381, 1.26316) -> (0.003381, 1.14316)
  circle A5 centre (-1.526619, 0.24316) radius 0.11
  circle A6 centre (-1.396619, 1.14316) radius 0.06
  circle A7 centre (-1.656619, 1.14316) radius 0.06
  line L13 (-1.776619, 1.26316) -> (-1.776619, -0.00684)
  circle A8 centre (-0.246619, 0.24316) radius 0.11
  point P0 (-7.3835, -1.47184)
  dimension "d63" = 1.78
  dimension "d64" = 1.27
  constraints: 28 end point, 9 centre point, 2 point on line
  measures "d63" distance of L10.start L0.start
  measures "d64" distance of L11.end L10.start
extrude "Extrusión16" cut sketch "Boceto19" against normal blind 15 contours L9 L8 L6 L5
sketch "Boceto20" plane through (1.486529, 1.47184, -4.497611) normal (0.8660254, 0, 0.5) x (0.5, 0, -0.8660254)
  line L0 (-0.172288, 0.983) -> (-0.312288, 0.983)
  line L1 (-0.312288, 0.683) -> (-0.172288, 0.683)
  line L2 (-0.172288, 0.683) -> (-0.172288, 0.983)
  circle A0 centre (-0.116619, 1.14316) radius 0.06
  line L3 (0.003381, 1.26316) -> (0.003381, 1.14316)
  line L4 (-0.312288, 0.983) -> (-0.312288, 0.683)
  line L5 (0.003381, -0.00684) -> (0.003381, 0.24316)
  circle A1 centre (-0.376619, 1.14316) radius 0.06
  circle A2 centre (-0.636619, 1.14316) radius 0.06
  circle A3 centre (-0.896619, 1.14316) radius 0.06
  line L6 (-0.76459, 0.802929) -> (-1.00459, 0.802929)
  circle A4 centre (-0.246619, 0.24316) radius 0.11
  line L7 (-0.76459, 0.352929) -> (-0.76459, 0.802929)
  line L8 (0.003381, 1.26316) -> (0.003381, -0.00684)
  circle A5 centre (-1.156619, 1.14316) radius 0.06
  line L9 (-1.00459, 0.352929) -> (-0.76459, 0.352929)
  line L10 (-1.00459, 0.802929) -> (-1.00459, 0.352929)
  line L11 (0.003381, 1.26316) -> (-1.776619, 1.26316)
  line L12 (-1.776619, -0.00684) -> (0.003381, -0.00684)
  line L13 (-1.776619, 1.26316) -> (-1.776619, -0.00684)
  circle A6 centre (-1.396619, 1.14316) radius 0.06
  circle A7 centre (-1.656619, 1.14316) radius 0.06
  circle A8 centre (-1.526619, 0.24316) radius 0.11
  point P0 (-4.638309, -1.47184)
  dimension "d67" = 1.78
  dimension "d68" = 1.27
  constraints: 28 end point, 9 centre point, 2 point on line
  measures "d67" distance of L12.start L5.start
  measures "d68" distance of L11.end L12.start
extrude "Extrusión17" cut sketch "Boceto20" against normal blind 15 contours L7 L9 L10 L6
sketch "Boceto21" plane through (0.043376, 1.465, 0.1) normal (1, 0, 0) x (0, 0, -1)
  line L0 (0.988309, 0.00684) -> (0.988309, 1.27)
  line L1 (0.976999, 0) -> (0.1, 0)
  line L2 (-0.02372, 0.359769) -> (-0.02372, 0.809769)
  line L3 (0.21628, 0.809769) -> (0.21628, 0.359769)
  line L4 (-0.02372, 0.809769) -> (0.21628, 0.809769)
  line L5 (0.21628, 0.359769) -> (-0.02372, 0.359769)
  circle A0 centre (0.738309, 0.25) radius 0.11
  circle A1 centre (-0.541691, 0.25) radius 0.11
  line L6 (-0.791691, 1.27) -> (-0.791691, 0)
  point P0 (0.1, -1.465)
  constraints: 14 end point, 2 centre point
extrude "Extrusión18" cut sketch "Boceto21" against normal blind 15 contours L2 L4 L3 L5
sketch "Boceto22" plane through (7.685812, 4.153752, 0.1) normal (0, 0, 1) x (0.8801071, -0.4747751, 0)
  arc A0 (-4.071533, 7.156173) -> (-6.735116, 4.499834) centre (1.277033, -0.870572) ccw
  line L0 (-6.735116, 4.499834) -> (-0.388836, 7.923345)
  arc A1 (-0.388836, 7.923345) -> (-4.071533, 7.156173) centre (-0.300845, -1.72176) ccw
  line L1 (-4.071533, 7.156173) -> (-3.561976, 6.21159)
  line L2 (-6.735116, 4.499834) -> (-0.388836, 7.923345)
  line L3 (-3.561976, 6.21159) -> (-6.735116, 4.499834)
  arc A2 (-4.071533, 7.156173) -> (-6.735116, 4.499834) centre (1.277033, -0.870572) ccw
  point P0 (-4.79224, -7.304779)
  constraints: 4 end point, 2 point on circle, 1 centre point, 1 midpoint, 1 perpendicular
revolve "Revolución2" add sketch "Boceto22" angle 180 about axis through (7.5, 12.385014, 0.1) along (0, -1, 0) contours L1 L0 A0
sketch "Boceto23" plane through (3.894598, 11.311754, 0.1) normal (0, 0, 1) x (1, 0, 0)
  arc A0 (3.605402, 1.07326) -> (0, 0) centre (4.501815, -8.530502) ccw
  line L0 (0, 0) -> (7.210804, 0)
  arc A1 (7.210804, 0) -> (3.605402, 1.07326) centre (2.70899, -8.530502) ccw
  arc A2 (7.210804, 0) -> (3.605402, 1.07326) centre (2.70899, -8.530502) ccw
  line L1 (7.210804, 0) -> (3.605402, 0)
  line L2 (0, 0) -> (7.210804, 0)
  line L3 (3.605402, 0.18663) -> (4.405402, 0.18663)
  line L4 (4.405402, 0.18663) -> (4.405402, 0.78663)
  line L5 (4.405402, 0.78663) -> (2.805402, 0.78663)
  line L6 (2.805402, 0.78663) -> (2.805402, 0.18663)
  line L7 (2.805402, 0.18663) -> (3.605402, 0.18663)
  point P0 (-3.894598, -11.311754)
  dimension "d75" = 0.8
  dimension "d76" = 0.6
  dimension "d77" = 1.6
  dimension "d78" = 0.6
  constraints: 12 end point, 2 perpendicular, 1 collinear, 1 midpoint, 1 point on line
  measures "d75" distance of L3.start L3.end
  measures "d76" distance of L3.end L4.end
  measures "d77" distance of L4.end L5.end
  measures "d78" distance of L5.end L6.end
extrude "Extrusión19" cut sketch "Boceto23" against normal blind 0.35 contours L7 L6 L5 L4 L3
sketch "Boceto24" plane through (7.5, 11.311754, 0.1) normal (0, -1, 0) x (1, 0, 0)
  line L0 (3.605402, 0) -> (-3.605402, 0)
  circle A0 centre (1.5, -0.8) radius 0.1
  circle A1 centre (-1.5, -0.8) radius 0.1
  point P0 (-7.5, -0.1)
  dimension "d125" = 0.2
  dimension "d126" = 0.2
  constraints: 2 centre point, 2 end point
  measures "d125" diameter of A1
  measures "d126" diameter of A0
extrude "Extrusión20" cut sketch "Boceto24" against normal blind 0.35
sketch "Boceto25" plane through (7.5, 11.311754, 0.1) normal (0, -1, 0) x (1, 0, 0)
  arc A0 (-3.605402, 0) -> (3.605402, 0) centre (0, 0) ccw
  circle A1 centre (-1.5, -0.8) radius 0.1
  circle A2 centre (1.5, -0.8) radius 0.1
  circle A3 centre (0, -2.450699) radius 0.075
  circle A4 centre (0, -1.850699) radius 0.075
  point P0 (-7.5, -0.1)
  dimension "d109" = 0.15
  dimension "d110" = 0.15
  constraints: 2 centre point, 1 other
  measures "d109" diameter of A3
  measures "d110" diameter of A4
extrude "Extrusión21" cut sketch "Boceto25" against normal blind 0.3 contours A3 | A4
sketch "Boceto26" plane through (7.685812, 4.153752, 0.1) normal (0, 0, 1) x (0.8801071, -0.4747751, 0)
  line L0 (-2.299378, -5.960001) -> (5.916505, -1.52793)
  line L1 (1.808563, -3.743966) -> (-1.380281, 1.110013)
  line L2 (7.72088, 1.110013) -> (8.165803, -0.314543)
  line L3 (-4.548676, -7.173388) -> (-5.494845, -6.01923)
  line L4 (8.165803, -0.314543) -> (7.989781, -0.409498)
  line L5 (7.989781, -0.409498) -> (7.484146, 0.527816)
  line L6 (7.484146, 0.527816) -> (7.842361, 0.721055)
  line L7 (8.165803, -0.314543) -> (7.842361, 0.721055)
  line L8 (7.72088, 1.110013) -> (8.165803, -0.314543)
  line L9 (1.808563, -3.743966) -> (-0.809923, 1.110013)
  line L10 (-5.236505, -6.334359) -> (-4.548676, -7.173388)
  line L11 (-4.548676, -7.173388) -> (-4.372655, -7.078433)
  line L12 (-4.372655, -7.078433) -> (-4.87829, -6.141119)
  line L13 (-4.87829, -6.141119) -> (-5.236505, -6.334359)
  line L14 (-4.548676, -7.173388) -> (-5.236505, -6.334359)
  line L15 (-5.236505, -6.334359) -> (-4.548676, -7.173388)
  line L16 (-5.236505, -6.334359) -> (-4.548676, -7.173388)
  line L17 (-4.548676, -7.173388) -> (-4.372655, -7.078433)
  line L18 (-4.79224, -7.304779) -> (8.409367, -0.183152)
  line L19 (-4.372655, -7.078433) -> (-4.87829, -6.141119)
  line L20 (-4.87829, -6.141119) -> (-5.236505, -6.334359)
  line L21 (7.484146, 0.527816) -> (7.989781, -0.409498)
  line L22 (7.989781, -0.409498) -> (8.165803, -0.314543)
  line L23 (8.165803, -0.314543) -> (7.842361, 0.721055)
  line L24 (7.842361, 0.721055) -> (7.484146, 0.527816)
  dimension "d111" = 0.2
  dimension "d112" = 1.065
  constraints: 40 end point, 5 collinear, 3 perpendicular, 3 symmetric about line, 1 midpoint, 1 point on line
  measures "d111" distance of L2.end L4.end
  measures "d112" distance of L4.end L5.end
extrude "Extrusión22" add sketch "Boceto26" against normal blind 1.1
sketch "Boceto27" plane through (14.523256, 0, 0.1) normal (-1, 0, 0) x (0, 0, 1)
  line L0 (-0.2, 0.852) -> (-0.2, 0.213)
  line L1 (-0.2, 0.852) -> (-0.86, 0.852)
  line L2 (-0.86, 0.213) -> (-0.86, 0.852)
  line L3 (-0.2, 0.213) -> (-0.86, 0.213)
  circle A0 centre (-0.5, 0.5325) radius 0.075
  point P0 (-0.1, 0)
  point P1 (-0.26, 0.213)
  dimension "d124" = 0.15
  constraints: 8 end point, 1 centre point
  measures "d124" diameter of A0
extrude "Extrusión23" cut sketch "Boceto27" against normal blind 0.4 contours A0
sketch "Boceto28" plane through (0.476744, 0, 0.1) normal (1, 0, 0) x (0, 0, -1)
  circle A0 centre (0.5, 0.5325) radius 0.075 projected
  point P0 (0.1, 0)
extrude "Extrusión24" cut sketch "Boceto28" against normal blind 0.4
sketch "Boceto29" plane through (3.894598, 11.311754, 0.1) normal (0, 0, 1) x (1, 0, 0)
  line L0 (0, 0) -> (7.210804, 0)
  line L1 (7.210804, 0) -> (-4.52187, 0)
  line L2 (-4.52187, 0) -> (-4.52187, 5.095282)
  line L3 (-4.52187, 5.095282) -> (13.689428, 5.095282)
  line L4 (13.689428, 5.095282) -> (13.689428, 0)
  line L5 (7.210804, 0) -> (13.689428, 0)
  line L6 (-0.044149, 0.249874) -> (7.254953, 0.249874)
  point P0 (-3.894598, -11.311754)
  constraints: 10 end point, 3 perpendicular, 1 horizontal, 1 parallel, 1 point on line
extrude "Extrusión25" cut sketch "Boceto29" against normal blind 10
sketch "Boceto30" plane through (7.5, 11.311754, 0) normal (0, 1, 0) x (1, 0, 0)
  arc A0 (3.605402, 0) -> (-3.605402, 0) centre (0, 0) ccw
  arc A1 (-0.669898, 4.042709) -> (0.669898, 4.042709) centre (0, 3.605402) ccw
  arc A2 (4.097836, 0) -> (-4.097836, 0) centre (0, 0) ccw
  arc A3 (0.669898, 4.042709) -> (-0.669898, 4.042709) centre (0, 0) ccw
  line L0 (0, 3.605402) -> (0, 3.205402)
  line L1 (0, 3.205402) -> (0.3, 3.205402)
  line L2 (0.3, 3.205402) -> (0.3, 3.805402)
  line L3 (0.3, 3.805402) -> (-0.3, 3.805402)
  line L4 (-0.3, 3.805402) -> (-0.3, 3.205402)
  line L5 (-0.3, 3.205402) -> (0, 3.205402)
  line L6 (-3.605402, -0.1) -> (-4.097836, -0.1)
  line L7 (-3.605402, 0) -> (-3.605402, -0.1)
  line L8 (-3.605402, -0.1) -> (-3.005402, -0.1)
  line L9 (-3.005402, -0.1) -> (-3.005402, 0.7)
  line L10 (-3.005402, 0.7) -> (-4.037606, 0.7)
  line L11 (-3.605402, -0.1) -> (-4.096616, -0.1)
  line L12 (-8.156048, -0.1) -> (-4.097836, -0.1)
  arc A4 (-4.037606, 0.7) -> (-4.096616, -0.1) centre (0, 0) ccw
  arc A5 (4.097836, 0) -> (-4.097836, 0) centre (0, 0) ccw
  line L13 (3.005402, -0.1) -> (3.005402, 0.7)
  line L14 (3.005402, 0.7) -> (4.037606, 0.7)
  arc A6 (4.096616, -0.1) -> (4.037606, 0.7) centre (0, 0) ccw
  line L15 (3.005402, -0.1) -> (4.096616, -0.1)
  line L16 (7.914206, -0.1) -> (3.605402, -0.1)
  line L17 (-3.005402, 0.3) -> (-3.355402, 0.3)
  line L18 (-3.355402, 0.3) -> (-3.355402, 0.5)
  line L19 (-3.355402, 0.5) -> (-3.755402, 0.5)
  line L20 (-3.755402, 0.5) -> (-3.755402, 0.1)
  line L21 (-3.755402, 0.1) -> (-3.355402, 0.1)
  line L22 (-3.355402, 0.1) -> (-3.355402, 0.3)
  line L23 (0, 0) -> (0, 1.219858)
  arc A7 (3.605402, 0) -> (-3.605402, 0) centre (0, 0) ccw
  line L24 (3.005402, 0.3) -> (3.355402, 0.3)
  line L25 (3.355402, 0.3) -> (3.355402, 0.5)
  line L26 (3.355402, 0.5) -> (3.755402, 0.5)
  line L27 (3.755402, 0.5) -> (3.755402, 0.1)
  line L28 (3.755402, 0.1) -> (3.355402, 0.1)
  line L29 (3.355402, 0.1) -> (3.355402, 0.3)
  point P0 (-7.5, 0)
  point P1 (-8.111288, -0.1)
  point P2 (7.874025, -0.1)
  dimension "d140" = 1.6
  dimension "d141" = 0.4
  dimension "d142" = 0.3
  dimension "d143" = 0.6
  dimension "d144" = 0.6
  dimension "d145" = 0.6
  dimension "d146" = 0.8
  dimension "d147" = 0.35
  dimension "d148" = 0.2
  dimension "d149" = 0.4
  dimension "d150" = 0.4
  dimension "d151" = 0.4
  constraints: 52 end point, 17 point on circle, 9 perpendicular, 8 symmetric about line, 6 centre point, 3 point on line, 2 collinear, 2 horizontal, 2 vertical, 1 concentric, 1 midpoint, 1 other
  measures "d140" diameter of A1
  measures "d141" distance of L0.start L0.end
  measures "d142" distance of L0.end L1.end
  measures "d143" distance of L1.end L2.end
  measures "d144" distance of L2.end L3.end
  measures "d145" distance of L6.start L8.end
  measures "d146" distance of L8.end L9.end
  measures "d147" distance of L17.start L17.end
  measures "d148" distance of L17.end L18.end
  measures "d149" distance of L18.end L19.end
  measures "d150" distance of L19.end L20.end
  measures "d151" distance of L20.end L21.end
extrude "Extrusión26" add sketch "Boceto30" against normal blind 0.25 contours L28 L27 L26 A0 L14 A2 A6 L15 L13 L24 L29 | L26 L25 L24 L13 L14 A0 | A1 A0 L4 L5 L1 L2 | A0 L2 L3 L4 A1 A2 | L10 L9 L17 L18 L19 A0 | A0 L19 L20 L21 L7 L6 A4 A2 L10 | L21 L22 L17 L9 L8 L7 A0
sketch "Boceto31" plane through (7.5, 11.311754, 0) normal (0, 1, 0) x (1, 0, 0)
  line L0 (-3.355402, 0.5) -> (-3.355402, 0.1)
  line L1 (-3.355402, 0.1) -> (-3.755402, 0.1)
  line L2 (-3.755402, 0.1) -> (-3.755402, 0.5)
  line L3 (-3.755402, 0.5) -> (-3.355402, 0.5)
  line L4 (-3.355402, 0.1) -> (-3.355402, 0.5)
  line L5 (-3.355402, 0.5) -> (-3.355402, 0.1)
  line L6 (3.355402, 0.1) -> (3.355402, 0.5)
  line L7 (3.355402, 0.5) -> (3.755402, 0.5)
  line L8 (3.755402, 0.5) -> (3.755402, 0.1)
  line L9 (3.755402, 0.1) -> (3.355402, 0.1)
  line L10 (3.355402, 0.1) -> (3.355402, 0.5)
  line L11 (0.3, 3.205402) -> (-0.3, 3.205402)
  line L12 (-0.3, 3.205402) -> (-0.3, 3.805402)
  line L13 (-0.3, 3.805402) -> (0.3, 3.805402)
  line L14 (0.3, 3.805402) -> (0.3, 3.205402)
  line L15 (0.3, 3.205402) -> (-0.3, 3.205402)
  point P0 (-7.5, 0)
  dimension "d154" = 0.4
  dimension "d155" = 0.4
  dimension "d156" = 0.4
  dimension "d157" = 0.4
  dimension "d158" = 0.6
  dimension "d159" = 0.6
  constraints: 24 end point, 3 perpendicular, 2 horizontal, 1 collinear, 1 vertical
  measures "d154" distance of L0.end L1.end
  measures "d155" distance of L1.end L2.end
  measures "d156" distance of L6.end L7.end
  measures "d157" distance of L7.end L8.end
  measures "d158" distance of L11.end L12.end
  measures "d159" distance of L12.end L13.end
extrude "Extrusión27" cut sketch "Boceto31" against normal blind 0.4
sketch "Boceto32" plane through (7.5, 11.061754, 0) normal (0, -1, 0) x (1, 0, 0)
  line L0 (-3.355402, -0.5) -> (-3.755402, -0.5)
  line L1 (-3.755402, -0.5) -> (-3.755402, -0.1)
  line L2 (-3.755402, -0.1) -> (-3.355402, -0.1)
  line L3 (-3.355402, -0.1) -> (-3.355402, -0.5)
  line L4 (-3.982775, -0.7) -> (-3.005402, -0.7)
  line L5 (-3.005402, -0.7) -> (-3.005402, 0.1)
  line L6 (-3.005402, 0.1) -> (-4.043822, 0.1)
  line L7 (0.3, -3.205402) -> (0.3, -3.805402)
  line L8 (0.3, -3.805402) -> (-0.3, -3.805402)
  line L9 (-0.3, -3.805402) -> (-0.3, -3.205402)
  line L10 (-0.3, -3.205402) -> (0.3, -3.205402)
  arc A0 (0.705962, -3.981723) -> (-0.705962, -3.981723) centre (0, -3.605402) ccw
  line L11 (3.355402, -0.5) -> (3.355402, -0.1)
  line L12 (3.355402, -0.1) -> (3.755402, -0.1)
  line L13 (3.755402, -0.1) -> (3.755402, -0.5)
  line L14 (3.755402, -0.5) -> (3.355402, -0.5)
  line L15 (3.005402, 0.1) -> (3.005402, -0.7)
  line L16 (3.005402, -0.7) -> (3.982775, -0.7)
  line L17 (4.043822, 0.1) -> (3.005402, 0.1)
  line L18 (-3.355402, -0.1) -> (-3.755402, -0.1)
  circle A1 centre (0, -3.505402) radius 0.1
  circle A2 centre (-3.555402, -0.3) radius 0.1
  circle A3 centre (3.555402, -0.3) radius 0.1
  line L19 (4.043822, 0.1) -> (4.043822, 0)
  arc A4 (3.982775, -0.7) -> (4.043822, 0) centre (0, 0) ccw
  arc A5 (-0.705962, -3.981723) -> (0.705962, -3.981723) centre (0, 0) ccw
  arc A6 (-4.043822, 0) -> (-3.982775, -0.7) centre (0, 0) ccw
  line L20 (-4.043822, 0) -> (-4.043822, 0.1)
  point P0 (-7.5, 0)
  dimension "d162" = 0.2
  dimension "d163" = 0.2
  dimension "d164" = 0.2
  constraints: 3 centre point
  measures "d162" diameter of A1
  measures "d163" diameter of A2
  measures "d164" diameter of A3
extrude "Extrusión28" add sketch "Boceto32" against normal blind 0.25 contours L0 L1 L2 L3 | L7 L8 L9 L10 | L11 L12 L13 L14
sketch "Boceto33" plane through (0, 2.735, 0) normal (0, 1, 0) x (1, 0, 0)
  line L0 (6.611691, 7.706624) -> (8.388309, 7.706624)
  line L1 (8.388309, 7.706624) -> (8.388309, 7.456624)
  line L2 (8.388309, 7.456624) -> (6.611691, 7.456624)
  line L3 (6.611691, 7.706624) -> (6.611691, 7.456624)
  line L4 (6.611691, 7.706624) -> (8.388309, 7.706624)
  line L5 (8.388309, 7.706624) -> (8.388309, 7.456624)
  line L6 (8.388309, 7.456624) -> (6.611691, 7.456624)
  line L7 (6.611691, 7.456624) -> (6.611691, 7.706624)
  line L8 (7.5, 7.456624) -> (7.5, 8.175896)
  line L9 (6.131323, 7.096637) -> (5.987048, 7.63508)
  line L10 (5.26199, 6.8637) -> (5.117715, 7.402143)
  line L11 (6.131323, 7.096637) -> (5.26199, 6.8637)
  line L12 (5.987048, 7.63508) -> (5.117715, 7.402143)
  circle A0 centre (5.624519, 7.24939) radius 0.1
  line L13 (9.73801, 6.8637) -> (9.882285, 7.402143)
  circle A1 centre (9.375481, 7.24939) radius 0.1
  line L14 (8.868677, 7.096637) -> (9.73801, 6.8637)
  line L15 (9.012952, 7.63508) -> (9.882285, 7.402143)
  line L16 (8.868677, 7.096637) -> (9.012952, 7.63508)
  line L17 (8.363785, 7.706624) -> (6.636215, 7.706624)
  line L18 (7.5, 7.706624) -> (6.823947, 8.246003)
  point P0 (0, 0)
  dimension "d171" = 0.25
  dimension "d172" = 0.2
  constraints: 36 end point, 2 centre point, 2 midpoint, 2 parallel, 2 perpendicular
  measures "d171" distance of L1.end L0.end
  measures "d172" diameter of A0
extrude "Extrusión29" add sketch "Boceto33" against normal blind 0.85 contours L11 L10 L12 L9 | L14 L16 L15 L13
sketch "Boceto34" plane through (0, 1.885, 0) normal (0, -1, 0) x (1, 0, 0)
  circle A0 centre (5.624519, -7.24939) radius 0.1
  circle A1 centre (9.375481, -7.24939) radius 0.1
  point P0 (0, 0)
extrude "Extrusión30" add sketch "Boceto34" against normal blind 0.35
